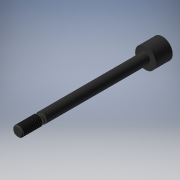
# Autodesk Inventor part: 4674228 DPDM-15---(r)
Saved by Autodesk Inventor 2019 (Build 230136000, 136)
## iProperties
Created: 2024-05-27
Part Number: 4674228 DPDM-15---(r)
Material: Generic
Catalog Web Link: www.cadenas.de
Description: DPDM(r)-Piston rod
Vendor: FESTO
Document SubType Name: Modeling
Designer: psAdmin
Manufacturer: FESTO
Mass: 0.403706 g
Surface Area: 5.06102 cm^2
Volume: 0.403706 cm^3
Density: 1 g/cm^3
Appearance: PSOLRGB-175-175-175
Category: PARTsolutions
Company: FESTO
Title: 4674228 DPDM-15---(r)
Author: Cadenas PARTsolutions
Comments: Piston rod
PSOL_IDENT_0: {$CADENAS_DATA/23d-libs/festo/parts/d/dpdm/parts/dpdm_rod.prj},201 {VTYP=3D},{NB=4674228 DPDM-15---(
PSOL_IDENT_1: r)},{LINA=4674228 DPDM-15---(r)},{NN=DPDM(r)},{DATE=23.02.2024 08:53:25},{GEOMDATE=23.02.2024 08:53:
PSOL_IDENT_2: 25},{VERSION=},{LINEID=10},{WBVAR=VER,HUB,FUN,KOT},{WBNUMERIC=HUB}  {NB=4674228 DPDM-15---(r)},{LINA=
PSOL_IDENT_3: 4674228 DPDM-15---(r)},{KT=DUMMY},{TNR=4674228},{TYP=DPDM},{KOL=6},{VER=-},{VERNB=},{HUB=15},{HUB1=5
PSOL_IDENT_4: ,10,15,20,25,30},{FUN=-},{FUN1='-','P','S'},{FUNNB=},{KOT=-},{KOT1='-','T'},{KOTNB=},{AM=7.000},{KK=
PSOL_IDENT_5: M3},{KKN=3.000},{WH=2.000},{MM=3.000},{SW=0.000},{LS=0.000},{ZJ=35.000},{ZM=37.000},{W22=0.000},{L2=
PSOL_IDENT_6: 33.000},{L4=42.000},{L5=9.000},{L6=0.000},{L8=44.000},{L1=19.35},{D8=0.000},{L9=0.000}
NB: 4674228 DPDM-15---(r)
NN: DPDM(r)
NT: Pirston rod
NBSYN: $TNR. $TYP.$VERNB.-$HUB.$FUNNB.$KOTNB.---(r)
LINA: 4674228 DPDM-15---(r)
CATALOG: Festo
TNR: 4674228
TYP: DPDM
KOL: 6
VER: -
HUB: 15
FUN: -
KOT: -
AM: 7
KK: M3
KKN: 3
WH: 2
MM: 3
SW: 0
LS: 0
ZJ: 35
ZM: 37
W22: 0
L2: 33
L4: 42
L5: 9
L6: 0
L8: 44
D8: 0
L9: 0
SUPPLIER: FESTO
ARTICLENO: 4674228 DPDM-15---(r)
BOMINFO: 4674228 DPDM-15---(r)
CREATOR: CADENAS GmbH
Autodesk Inventor part; units mm, degrees
sketch "Sketch_1" plane through (0, 0, 0) normal (1, 0, 0) x (0, 1, 0)
  line L0 (0, -35.65) -> (0, 0)
  line L1 (0, 0) -> (1.5, 0)
  line L2 (1.5, 0) -> (1.5, -30.65)
  line L3 (1.5, -30.65) -> (3, -30.65)
  line L4 (3, -30.65) -> (3, -35.65)
  line L5 (3, -35.65) -> (0, -35.65)
  line L6 (0, -35.65) -> (0, 0)
  constraints: 14 end point
revolve "Revolution1" add sketch "Sketch_1" angle 360 about axis through (0, 0, -35.65) along (0, 0, -1)
sketch "Sketch_2" plane through (0, 0, 0) normal (1, 0, 0) x (0, 1, 0)
  line L0 (0, 0) -> (0, 7)
  line L1 (0, 7) -> (1.1935, 7)
  line L2 (1.1935, 7) -> (1.5, 6.6935)
  line L3 (1.5, 6.6935) -> (1.5, 1.1111)
  line L4 (1.5, 1.1111) -> (1.0586, 0.6697)
  arc A0 (1.0586, 0.6697) -> (1, 0.5283) centre (1.2, 0.5283) ccw
  line L5 (1, 0.5283) -> (1, 0.2)
  arc A1 (1, 0.2) -> (1.2, 0) centre (1.2, 0.2) ccw
  line L6 (1.2, 0) -> (0, 0)
  line L7 (0, 0) -> (0, 7)
  constraints: 16 end point, 4 point on circle, 2 centre point
revolve "Revolution2" add sketch "Sketch_2" angle 360 about axis through (0, 0, 0) along (0, 0, -1)
thread "Thread1" size "M3x0.5" class "6g" standard "ISO Metric profile" full length
ref_plane "CP1_XY" through (0, 0, -35.65) normal (0, 0, -1) x (1, 0, 0)
ref_plane "CP1_YZ" through (0, 0, -35.65) normal (1, 0, 0) x (0, -1, 0)
ref_plane "CP1_ZX" through (0, 0, -35.65) normal (0, -1, 0) x (0, 0, -1)
ref_plane "CP_P_XY" through (0, 0, -35.65) normal (0, 0, 1) x (1, 0, 0)
ref_plane "CP_P_YZ" through (0, 0, -35.65) normal (1, 0, 0) x (0, 1, 0)
ref_plane "CP_P_ZX" through (0, 0, -35.65) normal (0, 1, 0) x (0, 0, 1)
ref_plane "CP_PL_XY" through (0, 0, 0) normal (0, 0, 1) x (1, 0, 0)
ref_plane "CP_PL_YZ" through (0, 0, 0) normal (1, 0, 0) x (0, 1, 0)
ref_plane "CP_PL_ZX" through (0, 0, 0) normal (0, 1, 0) x (0, 0, 1)
ref_plane "DIM_ZM_XY" through (0, 1.5, -67) normal (1, 0, 0) x (0, 0, -1)
ref_plane "DIM_ZM_YZ" through (0, 1.5, -67) normal (0, 0, -1) x (0, 1, 0)
ref_plane "DIM_ZM_ZX" through (0, 1.5, -67) normal (0, 1, 0) x (1, 0, 0)
ref_plane "NUT_6_10_T_1_XY" through (0, 0, -73) normal (0, 0, 1) x (1, 0, 0)
ref_plane "NUT_6_10_T_1_YZ" through (0, 0, -73) normal (1, 0, 0) x (0, 1, 0)
ref_plane "NUT_6_10_T_1_ZX" through (0, 0, -73) normal (0, 1, 0) x (0, 0, 1)
ref_plane "NUT_6_10_T_2_XY" through (0, 0, -71.2) normal (0, 0, 1) x (1, 0, 0)
ref_plane "NUT_6_10_T_2_YZ" through (0, 0, -71.2) normal (1, 0, 0) x (0, 1, 0)
ref_plane "NUT_6_10_T_2_ZX" through (0, 0, -71.2) normal (0, 1, 0) x (0, 0, 1)
ref_plane "NUT_CP_6_10_1_XY" through (0, 0, 5) normal (0, 0, 1) x (1, 0, 0)
ref_plane "NUT_CP_6_10_1_YZ" through (0, 0, 5) normal (1, 0, 0) x (0, 1, 0)
ref_plane "NUT_CP_6_10_1_ZX" through (0, 0, 5) normal (0, 1, 0) x (0, 0, 1)
ref_plane "NUT_CP_6_10_2_XY" through (0, 0, 3.2) normal (0, 0, 1) x (1, 0, 0)
ref_plane "NUT_CP_6_10_2_YZ" through (0, 0, 3.2) normal (1, 0, 0) x (0, 1, 0)
ref_plane "NUT_CP_6_10_2_ZX" through (0, 0, 3.2) normal (0, 1, 0) x (0, 0, 1)
body "Solid1"
